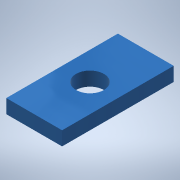
# Autodesk Inventor part: ADSK-MH-10043
Saved by Autodesk Inventor 2020.2 (Build 242310000, 310)
## iProperties
Created: 2008-03-10
Part Number: ADSK-MH-10043
Document SubType Name: Modeling
Designer: R.O'mahony
Density: 7.86 g/cm^3
Mass: 226.827 g
Surface Area: 88 cm^2
Volume: 28.8584 cm^3
Material: Steel, Mild
Description: Foot Support Plate
Appearance: Cyan
Engineer: Demir Ali
Checked By: Demir Ali
Company: Autodesk Ltd
Author: R.O'mahony
Keywords: Roller Conveyor
Revision Number: A
Autodesk Inventor part; units mm, degrees
ref_plane "YZ Plane" through (0, 0, 0) normal (1, 0, 0) x (0, 1, 0)
ref_plane "XZ Plane" through (0, 0, 0) normal (0, 1, 0) x (-1, 0, 0)
ref_plane "XY Plane" through (0, 0, 0) normal (0, 0, 1) x (1, 0, 0)
sketch "Sketch1" plane through (0, 0, 0) normal (0, 0, 1) x (1, 0, 0)
  circle A0 centre (2468.9202, -493.7243) radius 10
  line L0 (2488.9202, -533.7243) -> (2448.9202, -533.7243)
  line L1 (2448.9202, -533.7243) -> (2448.9202, -453.7243)
  line L2 (2448.9202, -453.7243) -> (2488.9202, -453.7243)
  line L3 (2488.9202, -533.7243) -> (2488.9202, -453.7243)
  point P0 (0, 0)
  point P1 (2456.4728, -559.596)
  point P2 (2456.4728, -563.8817)
  dimension "d1" = 40
  dimension "d3" = 80
  dimension "d5" = 40
  dimension "d8" = 20
  constraints: 8 end point, 1 centre point, 2 other
  measures "d1" distance of L2.end L1.end
  measures "d3" distance of L2.end L0.start
  measures "d5" vertical distance of L2.end A0.centre
  measures "d8" distance from line of A0.centre L1
extrude "Extrusion1" add sketch "Sketch1" along normal blind 10
body "Solid1"
